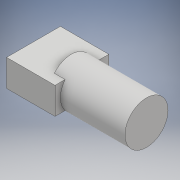
# Autodesk Inventor part: Union pie
Saved by Autodesk Inventor 2017 (Build 210142000, 142)
## iProperties
Part Number: Union pie
Material: Genérico
Document SubType Name: Modeling
Designer: HOME
Density: 1 g/cm^3
Appearance: Valor por defecto
Author: HOME
Autodesk Inventor part; units mm, degrees
ref_plane "YZ Plane" through (0, 0, 0) normal (1, 0, 0) x (0, 1, 0)
ref_plane "XZ Plane" through (0, 0, 0) normal (0, 1, 0) x (-1, 0, 0)
ref_plane "XY Plane" through (0, 0, 0) normal (0, 0, 1) x (1, 0, 0)
sketch "Boceto2" plane through (0, 0, 0) normal (1, 0, 0) x (0, 1, 0)
  circle A0 centre (0, 0) radius 4
  dimension "d3" = 8
  constraints: 1 centre point, 1 coincident
  measures "d3" diameter of A0
extrude "Extrusión2" add sketch "Boceto2" along normal blind 21
sketch "Boceto3" plane through (0, 0, 0) normal (-1, 0, 0) x (0, 0, 1)
  circle A0 centre (0, 0) radius 4 projected
  line L0 (-2.5, -5) -> (-2.5, 5)
  line L1 (-2.5, 5) -> (2.5, 5)
  line L2 (2.5, 5) -> (2.5, -5)
  line L3 (2.5, -5) -> (-2.5, -5)
  line L4 (-2.5, -5) -> (2.5, 5) construction
  line L5 (-2.5, 5) -> (2.5, -5) construction
  point P0 (-3.1225, 2.5)
  point P1 (-3.1225, -2.5)
  dimension "d15" = 10
  dimension "d16" = 5
  constraints: 12 end point, 2 horizontal, 2 midpoint, 2 point on circle, 2 vertical
  measures "d15" distance of L1.end L2.end
  measures "d16" distance of L0.end L1.end
extrude "Extrusión3" add sketch "Boceto3" against normal blind 9
sketch "Boceto4" plane through (0, 0, 0) normal (-1, 0, 0) x (0, 0, 1)
  line L0 (2.5, 3.1225) -> (2.5, -3.1225)
  line L1 (-2.5, 3.1225) -> (-2.5, -3.1225)
  line L2 (2.5, 5) -> (2.5, 3.1225) projected
  line L3 (-2.5, 3.1225) -> (-2.5, 5) projected
  arc A0 (2.5, -3.1225) -> (2.5, 3.1225) centre (0, 0) ccw
  arc A1 (-2.5, 3.1225) -> (-2.5, -3.1225) centre (0, 0) ccw
  constraints: 6 end point, 6 point on circle, 2 centre point, 2 collinear, 1 coincident
sketch "Boceto5" plane through (0, 0, 0) normal (-1, 0, 0) x (0, 0, 1)
  point P0 (0, 0)
extrude "Extrusión4" cut sketch "Boceto4" against normal blind 7
